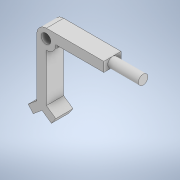
# Autodesk Inventor part: Hand 4
Saved by Autodesk Inventor 2021 (Build 250183000, 183)
## iProperties
Created: 2021-07-10
Part Number: Hand 4
Material: Generic
Document SubType Name: Modeling
Designer: Sampada S Kulkarni
Density: 1 g/cm^3
Appearance: Default
Author: Sampada S Kulkarni
Autodesk Inventor part; units mm, degrees
ref_plane "YZ Plane" through (0, 0, 0) normal (1, 0, 0) x (0, 1, 0)
ref_plane "XZ Plane" through (0, 0, 0) normal (0, 1, 0) x (-1, 0, 0)
ref_plane "XY Plane" through (0, 0, 0) normal (0, 0, 1) x (1, 0, 0)
sketch "Sketch1" plane through (0, 0, 0) normal (1, 0, 0) x (0, 1, 0)
  circle A0 centre (0, 0) radius 12.5
  dimension "d0" = 25
  constraints: 1 centre point, 1 coincident
  measures "d0" diameter of A0
extrude "Extrusion1" add sketch "Sketch1" along normal mid plane 80
sketch "Sketch2" plane through (0, 0, 0) normal (0, 0, 1) x (1, 0, 0)
  line L0 (-40, 12.5) -> (-40, -12.5) projected
  line L1 (-40, 12.5) -> (-190, 12.5)
  line L2 (-40, -12.5) -> (-165, -12.5)
  circle A0 centre (-190, -12.5) radius 25
  line L3 (-215, -12.5) -> (-215, -164.1266)
  line L4 (-190, -37.5) -> (-190, -162.5)
  line L5 (-190, -162.5) -> (-165.4254, -179.7073)
  line L6 (-190, -162.5) -> (-160, -162.5) construction
  line L7 (-165.4254, -179.7073) -> (-176.897, -196.0903)
  line L8 (-176.897, -196.0903) -> (-201.4715, -178.883)
  line L9 (-201.4715, -178.883) -> (-224.4529, -198.1667)
  line L10 (-224.4529, -198.1667) -> (-237.3086, -182.8458)
  line L11 (-237.3086, -182.8458) -> (-215, -164.1266)
  point P0 (0, 0)
  point P1 (-165, -12.5)
  dimension "d3" = 150
  dimension "d4" = 125
  constraints: 22 end point, 4 perpendicular, 3 horizontal, 2 point on circle, 2 tangent, 2 vertical, 1 centre point, 1 equal length
  measures "d3" distance of L0.start L1.end
  measures "d4" distance of L0.end L2.end
extrude "Extrusion2" add sketch "Sketch2" along normal mid plane 45
sketch "Sketch3" plane through (0, 0, -22.5) normal (0, 0, -1) x (-1, 0, 0)
  circle A0 centre (191.1384, -11.6978) radius 12.5
  point P0 (0, 0)
  constraints: 1 centre point
hole "Hole1" at (-191.1384, -11.6978, -22.5) direction (0, 0, 1) diameter 25 depth 45
body "Solid1"
